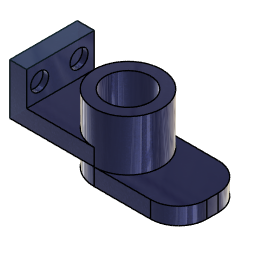
Exercise 9_ (Autodesk Fusion 360 design; units mm, degrees)
Autodesk Fusion 360 part; units mm, degrees
note: some values were not read from the file. Set by a fixed rule: which sketch regions a step uses.
sketch "Sketch1" plane through (0, 0, 0) normal (0, 1, 0) x (1, 0, 0)
  line L0 (0, 0) -> (0, -45)
  line L1 (0, -45) -> (15, -45)
  line L2 (15, -45) -> (15, -15)
  line L3 (15, -15) -> (75, -15)
  line L4 (75, -15) -> (75, 0)
  line L5 (75, 0) -> (0, 0)
  dimension "d1" = 45
  dimension "d2" = 15
  dimension "d3" = 30
  dimension "d4" = 60
  constraint coincident L0.start L5.end
  constraint vertical L0
  constraint perpendicular L0 L1
  constraint perpendicular L1 L2
  constraint perpendicular L2 L3
  constraint perpendicular L3 L4
  constraint perpendicular L0 L5
  measures "d1" distance of L0.start L0.end
  measures "d2" distance of L0.end L1.end
  measures "d3" distance of L1.end L2.end
  measures "d4" distance of L2.end L3.end
extrude "Extrude1" add sketch "Sketch1" along normal blind 60
sketch "Sketch2" plane through (15, 0, 0) normal (1, 0, 0) x (0, 1, 0)
  line L0 (0, 45) -> (0, 15)
  line L1 (0, 15) -> (60, 15)
  line L2 (60, 15) -> (60, 45)
  line L3 (60, 45) -> (0, 45)
  circle A0 centre (11.5393, 30) radius 8
  circle A1 centre (46.5393, 30) radius 8
  dimension "d7" = 15
  dimension "d8" = 15
  dimension "d9" = 35
  dimension "d10" = 16
  dimension "d11" = 16
  measures "d7" distance of L3 A0.centre
  measures "d8" distance of L3 A1.centre
  measures "d9" distance of A0.centre A1.centre
  measures "d10" diameter of A0
  measures "d11" diameter of A1
extrude "Extrude2" cut sketch "Sketch2" against normal blind 5 contours A0 | A1
sketch "Sketch3" plane through (0, 0, 15) normal (0, 0, 1) x (-1, 0, 0)
  line L0 (-15, 0) -> (-75, 0)
  line L1 (-75, 0) -> (-75, -60)
  line L2 (-75, -60) -> (-15, -60)
  line L3 (-15, -60) -> (-15, 0)
  line L4 (0, 0) -> (0, -30) construction
  line L5 (0, -30) -> (-75, -30) construction
  circle A0 centre (-75, -30) radius 30
  circle A1 centre (-75, -30) radius 20
  dimension "d14" = 30
  dimension "d15" = 75
  dimension "d16" = 60
  dimension "d17" = 40
  constraint coincident L4.start origin
  constraint vertical L4
  constraint perpendicular L4 L5
  constraint coincident L5.end A0.centre
  constraint concentric A0 A1
  measures "d14" distance of L4.start L4.end
  measures "d15" distance of L4.end L5.end
  measures "d16" diameter of A0
  measures "d17" diameter of A1
extrude "Extrude4" cut sketch "Sketch3" against normal blind 60 contours L1 A0 A1 | L1 A0 A1 | L1 A1 | L1 A1
extrude "Extrude5" add sketch "Sketch3" along normal blind 0 and the other way blind 15 contours L1 A0 A1 | L1 A0 A1
extrude "Extrude6" add sketch "Sketch3" against normal blind 15 from surface at -15 contours L1 A0 A1 | L1 A0 A1
extrude "Extrude7" add sketch "Sketch3" along normal blind 30 contours L1 A0 A1 | L1 A0 A1
sketch "Sketch4" plane through (0, 0, 0) normal (0, -1, 0) x (1, 0, 0)
  line L0 (0, 0) -> (75, 0)
  line L1 (75, 0) -> (75, 15)
  line L2 (75, 15) -> (15, 15)
  line L3 (15, 15) -> (15, 45)
  line L4 (15, 45) -> (0, 45)
  line L5 (0, 45) -> (0, 0)
sketch "Sketch5" plane through (0, 0, 45) normal (0, 0, 1) x (-1, 0, 0)
  circle A0 centre (-75, -30) radius 20
  circle A1 centre (-75, -30) radius 30
sketch "Sketch6" plane through (0, 0, 0) normal (-1, 0, 0) x (0, -1, 0)
  line L0 (0, 0) -> (0, 45)
  line L1 (0, 45) -> (-60, 45)
  line L2 (-60, 45) -> (-60, 0)
  line L3 (-60, 0) -> (0, 0)
sketch "Sketch7" plane through (0, 0, 0) normal (-1, 0, 0) x (0, -1, 0)
sketch "Sketch8" plane through (0, 0, 0) normal (0, -1, 0) x (1, 0, 0)
sketch "Sketch9" plane through (0, 0, 45) normal (0, 0, 1) x (-1, 0, 0)
sketch "Sketch10" plane through (0, 0, 0) normal (0, 0, -1) x (1, 0, 0)
  arc A0 (75, 0) -> (75, -60) centre (75, -30) ccw
  line L0 (75, 0) -> (0, 0)
  line L1 (0, 0) -> (0, -60)
  line L2 (0, -60) -> (75, -60)
  circle A1 centre (75, -30) radius 30
  circle A2 centre (75, -30) radius 20
  line L3 (75, 0) -> (150, 0)
  line L4 (150, 0) -> (150, -60)
  line L5 (150, -60) -> (75, -60)
  constraint coincident A0.start L0.start
  constraint tangent A1 L3
  constraint parallel L0 L3
  constraint perpendicular L2 L4
  constraint coincident A0.end L2.end
  constraint tangent A0 L5
extrude "Extrude8" add sketch "Sketch10" along normal blind 15 contours A1 L3 L4 L5
fillet "Fillet1" radius 25 2 edges at (150, 60, -7.5) (150, 0, -7.5)
sketch "Sketch11" plane through (0, 0, 45) normal (0, 0, 1) x (-1, 0, 0)
  line L0 (0, 0) -> (-15, 0)
  line L1 (-15, 0) -> (-15, -60)
  line L2 (-15, -60) -> (0, -60)
  line L3 (0, -60) -> (0, 0)
